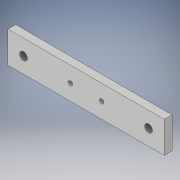
# Autodesk Inventor part: Plate that doewsn't touch lander
Saved by Autodesk Inventor 2019 (Build 230136000, 136)
## iProperties
Created: 2019-02-14
Part Number: Plate that doewsn't touch lander
Material: Generic
Document SubType Name: Modeling
Designer: Delta
Density: 1 g/cm^3
Appearance: Default
Author: Delta
Autodesk Inventor part; units mm, degrees
ref_plane "YZ Plane" through (0, 0, 0) normal (1, 0, 0) x (0, 1, 0)
ref_plane "XZ Plane" through (0, 0, 0) normal (0, 1, 0) x (-1, 0, 0)
sketch "Sketch1" plane through (0, 0, 0) normal (0, 0, 1) x (1, 0, 0)
  line L0 (0, 0) -> (127, 0)
  line L1 (127, 0) -> (127, 25.4)
  line L2 (127, 25.4) -> (0, 25.4)
  line L3 (0, 25.4) -> (0, 0)
  dimension "d0" = 127
  dimension "d1" = 25.4
  constraints: 8 end point, 2 parallel, 1 horizontal, 1 perpendicular
  measures "d0" distance of L2.end L1.end
  measures "d1" distance of L1.end L0.end
extrude "Extrusion1" add sketch "Sketch1" along normal blind 6.35
sketch "Sketch2" plane through (0, 0, 6.35) normal (0, 0, 1) x (1, 0, 0)
  line L0 (0, 25.4) -> (0, 0) projected
  point P0 (12.7, 12.7)
  dimension "d4" = 12.7
  measures "d4" distance from line of point (12.7, 12.7) L0
hole "Hole1" at (12.7, 12.7, 6.35) direction (0, 0, -1) diameter 6.35 end through all
thread "Thread1" size "1/4-20 UNC" class "2B" standard "ANSI Unified Screw Threads" full length
ref_plane "Work Plane1" through (63.5, 0, 0) normal (1, 0, 0) x (0, 0, -1)
mirror "Mirror1" about plane through (63.5, 0, 0) normal (1, 0, 0) of "Hole1"
thread "Thread2" size "1/4-20 UNC" class "2B" standard "ANSI Unified Screw Threads" full length
sketch "Sketch4" plane through (0, 0, 6.35) normal (0, 0, 1) x (1, 0, 0)
  line L0 (127, 25.4) -> (0, 25.4) projected
  line L1 (0, 25.4) -> (0, 0) projected
  line L2 (127, 0) -> (127, 25.4) projected
  circle A0 centre (50.8, 12.7) radius 1.778
  circle A1 centre (76.2, 12.7) radius 1.778
  dimension "d28" = 12.7
  dimension "d29" = 12.7
  dimension "d30" = 50.8
  dimension "d31" = 50.8
  dimension "d32" = 3.556
  constraints: 2 centre point, 2 coincident
  measures "d28" distance from line of L0 point (50.8, 12.7)
  measures "d29" distance from line of L0 point (76.2, 12.7)
  measures "d30" distance from line of L1 point (50.8, 12.7)
  measures "d31" distance from line of L2 point (76.2, 12.7)
  measures "d32" diameter of A0
extrude "Extrusion3" cut sketch "Sketch4" against normal blind 6.35
equation "\"d29\" = d28"
equation "\"d31\" = d30"
body "Solid1"
